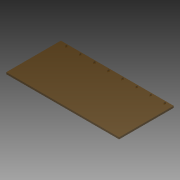
# Autodesk Inventor part: case_door
Saved by Autodesk Inventor 2014 (Build 180170000, 170)
## iProperties
Created: 2013-08-29
Part Number: case_door
Material: Polycarbonate, Smoke
Document SubType Name: Modeling
Designer: Edward
Density: 1.2 g/cm^3
Appearance: Polycarbonate - Smoked
Author: Edward
Autodesk Inventor part; units mm, degrees
ref_plane "YZ Plane" through (0, 0, 0) normal (1, 0, 0) x (0, 1, 0)
ref_plane "XZ Plane" through (0, 0, 0) normal (0, 1, 0) x (-1, 0, 0)
ref_plane "XY Plane" through (0, 0, 0) normal (0, 0, 1) x (1, 0, 0)
sketch "Sketch1" plane through (0, 0, 0) normal (0, 0, 1) x (1, 0, 0)
  line L0 (-203.65, 98.5) -> (203.65, 98.5)
  line L1 (203.65, 98.5) -> (203.65, -98.5)
  line L2 (203.65, -98.5) -> (-203.65, -98.5)
  line L3 (-203.65, -98.5) -> (-203.65, 98.5)
  point P0 (0, 0)
  dimension "d0" = 407.3
  dimension "d1" = 197
  dimension "d2" = 203.65
  dimension "d3" = 98.5
  constraints: 8 end point, 2 parallel, 1 horizontal, 1 perpendicular
  measures "d0" distance of L1.end L2.end
  measures "d1" distance of L0.end L1.end
  measures "d2" distance from line of L3 point (0, 0)
  measures "d3" distance from line of L0 point (0, 0)
extrude "Extrusion1" add sketch "Sketch1" along normal blind 6.35
sketch "Sketch2" plane through (0, 0, 6.35) normal (0, 0, 1) x (1, 0, 0)
  line L0 (203.65, 98.5) -> (-203.65, 98.5) projected
  line L1 (-203.65, 98.5) -> (-203.65, -98.5) projected
  line L2 (-177.8, 93.65) -> (-177.8, 90.65) construction
  line L3 (-179.55, 93.65) -> (-179.55, 90.65)
  line L4 (-176.05, 90.65) -> (-176.05, 93.65)
  arc A0 (-176.05, 93.65) -> (-179.55, 93.65) centre (-177.8, 93.65) ccw
  arc A1 (-179.55, 90.65) -> (-176.05, 90.65) centre (-177.8, 90.65) ccw
  point P0 (0, 0)
  point P1 (-177.8, 92.15)
  dimension "d7" = 3
  dimension "d8" = 3.5
  dimension "d9" = 25.85
  dimension "d10" = 6.35
  constraints: 8 end point, 4 point on circle, 4 tangent, 2 centre point, 2 parallel, 1 midpoint
  measures "d7" distance of L2.start L2.end
  measures "d8" diameter of A1
  measures "d9" distance from line of L1 point (-177.8, 92.15)
  measures "d10" distance from line of L0 point (-177.8, 92.15)
extrude "Extrusion2" cut sketch "Sketch2" against normal through all
pattern_linear "Rectangular Pattern1" count 8 spacing 50.8 along (1, 0, 0) of "Extrusion2"
equation "\"d2\" = 0.5 * d0"
equation "\"d3\" = 0.5 * d1"
body "Solid1"
